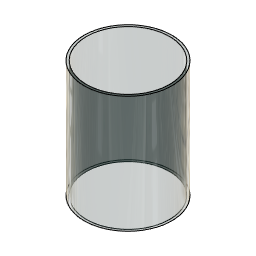
Lantern (Autodesk Fusion 360 archive; units mm, degrees)
design "BottleGlas"
Autodesk Fusion 360 part; units mm, degrees
sketch "Skizze1" plane through (0, 0, 0) normal (0, 0, 1) x (1, 0, 0)
  circle A0 centre (0, 0) radius 30
  circle A1 centre (0, 0) radius 28.45
  dimension "d1" = 60
  dimension "d2" = 56.9
  constraint coincident A0.centre A1.centre
  measures "d1" diameter of A0
  measures "d2" diameter of A1
extrude "Extrusion1" add sketch "Skizze1" along normal blind 80
equation "d2 = 60 mm - 3.1 mm"
